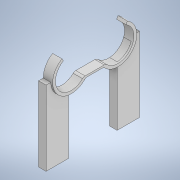
# Autodesk Inventor part: ultrasonic_fastening
Saved by Autodesk Inventor 2022 (Build 260153000, 153)
## iProperties
Created: 2022-02-09
Part Number: ultrasonic_fastening
Material: Generic
Document SubType Name: Modeling
Designer: Iñigo
Density: 1 g/cm^3
Appearance: Default
Author: Iñigo
Autodesk Inventor part; units mm, degrees
ref_plane "YZ Plane" through (0, 0, 0) normal (1, 0, 0) x (0, 1, 0)
ref_plane "XZ Plane" through (0, 0, 0) normal (0, 1, 0) x (-1, 0, 0)
sketch "Sketch3" plane through (0, 0, 0) normal (1, 0, 0) x (0, 1, 0)
  arc A0 (7.6059, 16.7425) -> (-5.7973, 6.5139) centre (0.2447, 12.4925) ccw
  arc A1 (8.905, 17.4925) -> (-6.7785, 5.374) centre (0.2447, 12.4925) ccw
  line L0 (8.7447, -0.0075) -> (4.3518, -0.0075)
  line L1 (0.2447, 12.4925) -> (0.2447, 2.4925) construction
  line L2 (0.2447, 12.4925) -> (0.2447, 2.4925) construction
  line L3 (8.905, 17.4925) -> (7.6059, 16.7425)
  arc A2 (-6.7785, -5.3889) -> (8.905, -17.5075) centre (0.2447, -12.5075) ccw
  arc A3 (-5.7973, -6.5288) -> (7.6059, -16.7575) centre (0.2447, -12.5075) ccw
  line L4 (8.905, -17.5075) -> (7.6059, -16.7575)
  line L5 (-5.219, 5.1072) -> (-5.219, -5.1221)
  line L6 (-6.1832, 3.9502) -> (-6.1832, -3.9652)
  arc A4 (-5.219, 5.1072) -> (-5.7973, 6.5139) centre (-7.219, 5.1072) ccw
  arc A5 (-5.7973, -6.5288) -> (-5.219, -5.1221) centre (-7.219, -5.1221) ccw
  arc A6 (-6.1832, 3.9502) -> (-6.7785, 5.374) centre (-8.1832, 3.9502) ccw
  arc A7 (-6.7785, -5.3889) -> (-6.1832, -3.9652) centre (-8.1832, -3.9652) ccw
  point P0 (0, 0)
  point P1 (0.2447, -0.2026)
  point P2 (-6.1832, 4.8321)
  point P3 (-6.1832, -4.847)
  point P4 (-5.219, -5.9961)
  point P5 (-6.1832, -4.847)
  dimension "d18" = 20
  dimension "d19" = 12.5
  dimension "d20" = 2
  dimension "d21" = 2
  constraints: 18 point on circle, 14 end point, 8 centre point, 8 tangent, 5 symmetric about line, 3 point on line, 2 coincident, 2 equal radius, 2 other
  measures "d18" diameter of A1
  measures "d19" distance from line of A0.centre L0
  measures "d20" radius of A4
  measures "d21" radius of A6
extrude "Extrusion3" add sketch "Sketch3" along normal blind 5
ref_plane "Work Plane3" through (0, 0, 22) normal (0, 0, 1) x (1, 0, 0)
sketch "Sketch4" plane through (0, 0, 22) normal (0, 0, 1) x (1, 0, 0)
  line L0 (0, 0) -> (4, 0)
  line L1 (4, 0) -> (4, -40)
  line L2 (4, -40) -> (0, -40)
  line L3 (0, -40) -> (0, 0)
  dimension "d26" = 40
  constraints: 8 end point, 2 parallel, 1 horizontal, 1 perpendicular
  measures "d26" distance of L0.end L1.end
extrude "Extrusion4" add sketch "Sketch4" along normal blind 3
sketch "Sketch5" plane through (0, 0, 22) normal (0, 0, -1) x (-1, 0, 0)
  line L0 (0, -8.2553) -> (0, 7.6059) projected
  line L1 (-4, -40) -> (0, -40)
  line L2 (0, -40) -> (0, -2.5366)
  line L3 (0, -2.5366) -> (-4, -2.5366)
  line L4 (-4, -2.5366) -> (-4, -40)
  point P0 (0, 0)
  point P1 (0, -5.7973)
  constraints: 8 end point, 2 parallel, 1 horizontal, 1 perpendicular, 1 point on line
extrude "Extrusion5" add sketch "Sketch5" along normal blind 9
sketch "Sketch6" plane through (4, -8.2401, 13) normal (1, 0, 0) x (0, 0, -1)
  line L0 (-7.5246, 5.7036) -> (0, 5.7036) projected
  line L1 (0, 5.7036) -> (0, 0) projected
  arc A0 (0, 0) -> (6.4861, 2.4428) centre (0.5075, 8.4848) ccw projected
  arc A1 (-7.5246, 5.7036) -> (0, 0) centre (0.5075, 8.4848) ccw
  line L2 (-7.5246, 5.7036) -> (0, 5.7036)
  line L3 (0, 0) -> (0, 5.7036)
  point P0 (13, 8.2401)
  constraints: 4 end point, 2 collinear, 2 point on circle, 1 centre point
extrude "Extrusion6" cut sketch "Sketch6" against normal blind 4
mirror "Mirror1" about plane through (0, 0, 0) normal (0, 0, 1) of "Extrusion4", "Extrusion5", "Extrusion6"
body "Solid2"
